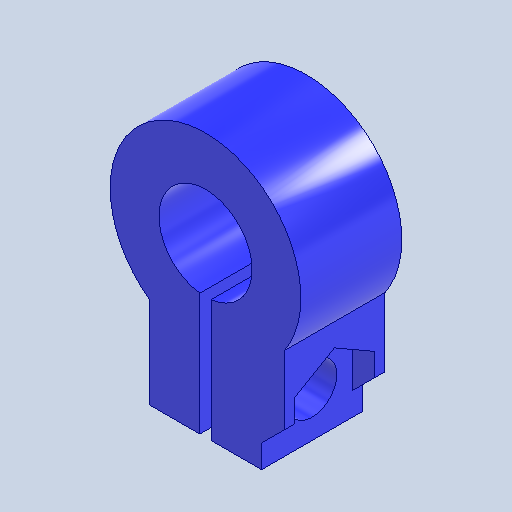
# Autodesk Inventor part: 軸止め
Saved by Autodesk Inventor 2022 (Build 260153000, 153)
## iProperties
Created: 2019-12-20
Part Number: 軸止め
Material: ABS プラスチック
Document SubType Name: Modeling
Designer: Hagihara Yuya
Density: 1.06 g/cm^3
Appearance: 青 - 壁塗料 - 光沢
Mass: 1.99053 g
Surface Area: 15.3185 cm^2
Volume: 1.87786 cm^3
Author: Hagihara Yuya
Autodesk Inventor part; units mm, degrees
ref_plane "YZ Plane" through (0, 0, 0) normal (1, 0, 0) x (0, 1, 0)
ref_plane "XZ Plane" through (0, 0, 0) normal (0, 1, 0) x (-1, 0, 0)
ref_plane "XY Plane" through (0, 0, 0) normal (0, 0, 1) x (1, 0, 0)
sketch "スケッチ1" plane through (0, 0, 0) normal (0, 0, 1) x (1, 0, 0)
  line L0 (0, 0) -> (10, 0)
  line L1 (10, 0) -> (10, 15)
  line L2 (10, 15) -> (0, 15)
  line L3 (0, 15) -> (0, 0)
  circle A0 centre (5, 15) radius 8.5
  point P0 (0, 8.1261)
  point P1 (10, 8.1261)
  dimension "d0" = 15
  dimension "d1" = 17
  dimension "d27" = 10
  dimension "d28" = 5
  constraints: 8 end point, 2 parallel, 1 centre point, 1 horizontal, 1 midpoint, 1 perpendicular
  measures "d0" distance of L2.end L0.start
  measures "d1" diameter of A0
  measures "d27" distance of L1.end L2.end
  measures "d28" distance of A0.centre L2.end
extrude "押し出し1" add sketch "スケッチ1" along normal blind 9
sketch "スケッチ2" plane through (0, 0, 9) normal (0, 0, 1) x (1, 0, 0)
  arc A0 (10, 8.1261) -> (0, 8.1261) centre (5, 15) ccw projected
  point P0 (0, 0)
  constraints: 1 coincident
hole "穴1" at (5, 15, 9) direction (0, 0, -1) diameter 8.3 end through all
sketch "スケッチ3" plane through (0, 0, 9) normal (0, 0, 1) x (1, 0, 0)
  line L0 (0, 0) -> (10, 0) projected
  line L1 (4.5, 0) -> (5.5, 0)
  line L2 (5.5, 0) -> (5.5, 15)
  line L3 (5.5, 15) -> (4.5, 15)
  line L4 (4.5, 15) -> (4.5, 0)
  line L5 (0, 8.1261) -> (0, 0) projected
  circle A0 centre (5, 15) radius 4.15 projected
  point P0 (5, 0)
  point P1 (5, 0)
  dimension "d14" = 1
  constraints: 8 end point, 3 midpoint, 2 coincident, 2 parallel, 1 horizontal, 1 perpendicular, 1 point on line
  measures "d14" distance of L2.end L3.end
extrude "押し出し2" cut sketch "スケッチ3" against normal up to surface (9 mm away) contours L4 A0 L2 L0 | L4 L3 L2 A0 picked at (4.9443, 13.6178)
sketch "スケッチ4" plane through (10, 0, 0) normal (1, 0, 0) x (0, 0, -1)
  circle A0 centre (-4.5, 4) radius 1.5
  line L0 (0, 0) -> (-9, 0) projected
  line L1 (0, 0) -> (0, 8.1261) projected
  line L2 (-4.5, 0) -> (-4.5, 10)
  point P0 (0, 10)
  dimension "d17" = 4
  dimension "d19" = 3
  constraints: 2 end point, 1 centre point, 1 midpoint, 1 point on line, 1 vertical
  measures "d17" distance from line of L0 A0.centre
  measures "d19" diameter of A0
hole "穴2" at (10, 4, 4.5) direction (-1, 0, 0) diameter 4.4 end through all
sketch "スケッチ7" plane through (10, 0, 0) normal (1, 0, 0) x (0, 0, -1)
  circle A0 centre (-4.5, 4) radius 2.2 projected
  line L0 (-4.5, 8.1569) -> (-0.9, 6.0785)
  line L1 (-0.9, 6.0785) -> (-0.9, 1.9215)
  line L2 (-0.9, 1.9215) -> (-4.5, -0.1569)
  line L3 (-4.5, -0.1569) -> (-8.1, 1.9215)
  line L4 (-8.1, 1.9215) -> (-8.1, 6.0785)
  line L5 (-8.1, 6.0785) -> (-4.5, 8.1569)
  line L6 (-9, 10.8802) -> (-9, 0) projected
  line L7 (0, 0) -> (0, 8.1261) projected
  line L8 (-9, 10.8802) -> (0, 10.8802)
  line L9 (0, 10.8802) -> (0, 4.0631)
  line L10 (0, 4.0631) -> (-9, 4.0631)
  line L11 (-9, 4.0631) -> (-9, 10.8802)
  point P0 (-4.5, 4)
  point P1 (-0.9, 4.0631)
  point P2 (-8.1, 4.0631)
  dimension "d35" = 7.2
  constraints: 20 end point, 2 parallel, 1 coincident, 1 horizontal, 1 horizontal alignment, 1 midpoint, 1 perpendicular, 13 other
  measures "d35" distance between parallel lines of L0 L3
extrude "押し出し5" add sketch "スケッチ7" along normal blind 2 contours L1 L0 L5 L4 L10 L6 L8 L9 L7
chamfer "面取り1" distance 2 angle 45 2 edges at (10, 4.0631, 8.55) (10, 4.0631, 0.45)
equation "\"d28\" = 0.5 * d27"
